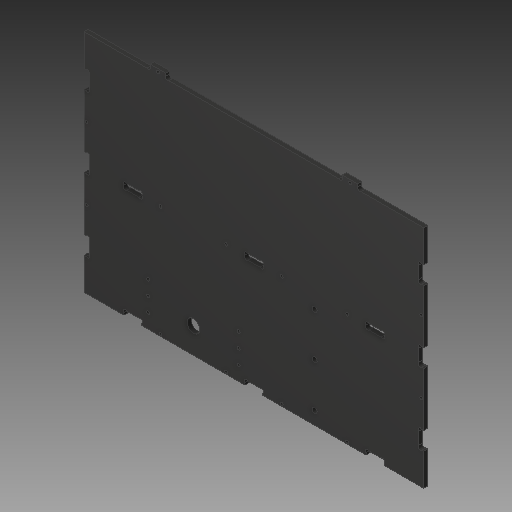
# Autodesk Inventor part: BA02
Saved by Autodesk Inventor 2017 (Build 210142000, 142)
## iProperties
Created: 2019-05-22
Part Number: BA02
Material: Polyethylene, High Density
Document SubType Name: Modeling
Designer: Dell
Density: 0.952 g/cm^3
Appearance: Smooth - Black
Mass: 1090.28 g
Surface Area: 3771.88 cm^2
Volume: 1145.26 cm^3
Author: Dell
Autodesk Inventor part; units mm, degrees
ref_plane "YZ Plane" through (0, 0, 0) normal (1, 0, 0) x (0, 1, 0)
ref_plane "XZ Plane" through (0, 0, 0) normal (0, 1, 0) x (-1, 0, 0)
ref_plane "XY Plane" through (0, 0, 0) normal (0, 0, 1) x (1, 0, 0)
sketch "Sketch1" plane through (0, 0, 0) normal (0, 0, 1) x (1, 0, 0)
  line L0 (0, 0) -> (525.78, 0)
  line L1 (525.78, 0) -> (525.78, 349.25)
  line L2 (525.78, 349.25) -> (0, 349.25)
  line L3 (0, 349.25) -> (0, 0)
  line L4 (239.14, 66.95) -> (239.14, 21.95) construction
  circle A0 centre (239.14, 66.95) radius 2.3813
  circle A1 centre (239.14, 21.95) radius 2.3813
  circle A2 centre (239.14, 44.45) radius 2.3813
  line L5 (179.14, 29.45) -> (179.14, 49.45) construction
  line L6 (169.14, 66.95) -> (169.14, 21.95) construction
  line L7 (179.14, 49.45) -> (159.14, 49.45) construction
  line L8 (159.14, 29.45) -> (179.14, 29.45) construction
  circle A3 centre (169.14, 39.45) radius 10
  line L9 (239.14, 21.95) -> (99.14, 21.95) construction
  line L10 (99.14, 66.95) -> (239.14, 66.95) construction
  line L11 (99.14, 44.45) -> (239.14, 44.45) construction
  line L12 (159.14, 49.45) -> (159.14, 29.45) construction
  line L13 (0, 0) -> (525.78, 0) construction
  line L14 (525.78, 0) -> (525.78, 88.9)
  line L15 (525.78, 88.9) -> (0, 88.9) construction
  line L16 (0, 88.9) -> (0, 0) construction
  line L17 (99.14, 21.95) -> (99.14, 66.95) construction
  circle A4 centre (99.14, 66.95) radius 2.3812
  circle A5 centre (99.14, 21.95) radius 2.3812
  circle A6 centre (99.14, 44.45) radius 2.3812
  point P0 (179.14, 39.45)
  point P1 (159.14, 39.45)
  point P2 (0, 44.45)
  dimension "d0" = 349.25
  dimension "d1" = 525.78
  dimension "d2" = 45
  dimension "d3" = 140
  dimension "d4" = 4.7625
  dimension "d5" = 4.7625
  dimension "d6" = 4.7625
  dimension "d7" = 4.7625
  dimension "d8" = 4.7625
  dimension "d9" = 4.7625
  dimension "d10" = 60
  dimension "d11" = 7.5
  dimension "d12" = 20
  dimension "d13" = 20
  dimension "d15" = 88.9
  dimension "d78" = 169.14
  dimension "d79" = 39.45
  constraints: 36 end point, 8 parallel, 7 midpoint, 6 centre point, 5 coincident, 4 perpendicular, 3 horizontal alignment, 2 horizontal, 2 point on line, 2 other
  measures "d0" distance of L2.end L0.start
  measures "d1" distance of L0.start L0.end
  measures "d2" distance of L4.start L4.end
  measures "d3" distance of L17.end L4.start
  measures "d4" diameter of A4
  measures "d5" diameter of A6
  measures "d6" diameter of A5
  measures "d7" diameter of A1
  measures "d8" diameter of A2
  measures "d9" diameter of A0
  measures "d10" distance from line of L11.end L5
  measures "d11" distance between parallel lines of L9 L8
  measures "d12" distance of L5.end L12.start
  measures "d13" distance of L12.start L8.start
  measures "d15" distance of L15.end L13.start
  measures "d78" distance from line of L3 point (169.14, 39.45)
  measures "d79" distance from line of L0 point (169.14, 39.45)
extrude "Extrusion1" add sketch "Sketch1" along normal blind 6.35
sketch "Sketch2" plane through (0, 0, 6.35) normal (0, 0, 1) x (1, 0, 0)
  line L0 (525.78, 349.25) -> (0, 349.25) projected
  line L1 (101.6, 349.25) -> (127, 349.25)
  line L2 (127, 349.25) -> (127, 355.6)
  line L3 (127, 355.6) -> (101.6, 355.6)
  line L4 (101.6, 355.6) -> (101.6, 349.25)
  line L5 (0, 349.25) -> (0, 0) projected
  line L6 (262.89, 349.25) -> (262.89, 386.8153)
  line L7 (0, 349.25) -> (525.78, 349.25)
  line L8 (424.18, 349.25) -> (398.78, 349.25)
  line L9 (398.78, 349.25) -> (398.78, 355.6)
  line L10 (398.78, 355.6) -> (424.18, 355.6)
  line L11 (424.18, 355.6) -> (424.18, 349.25)
  dimension "d18" = 25.4
  dimension "d19" = 6.35
  dimension "d20" = 101.6
  constraints: 20 end point, 6 symmetric about line, 2 parallel, 2 point on line, 1 horizontal, 1 midpoint, 1 perpendicular, 1 vertical
  measures "d18" distance of L3.end L2.end
  measures "d19" distance of L2.end L1.end
  measures "d20" distance from line of L5 L3.end
extrude "Extrusion2" add sketch "Sketch2" against normal blind 6.35
sketch "Sketch3" plane through (0, 0, 6.35) normal (0, 0, 1) x (1, 0, 0)
  line L0 (101.6, 355.6) -> (101.6, 349.25) projected
  line L1 (127, 355.6) -> (101.6, 355.6) projected
  line L2 (424.18, 355.6) -> (424.18, 349.25) projected
  line L3 (398.78, 355.6) -> (424.18, 355.6) projected
  circle A0 centre (114.3, 352.425) radius 2.25
  circle A1 centre (411.48, 352.425) radius 2.25
  point P0 (0, 0)
  point P1 (114.3, 355.6)
  point P2 (101.6, 352.425)
  point P3 (424.18, 352.425)
  point P4 (411.48, 355.6)
  dimension "d23" = 4.5
  dimension "d24" = 4.5
  constraints: 4 midpoint, 2 centre point, 2 horizontal alignment, 2 vertical alignment
  measures "d23" diameter of A0
  measures "d24" diameter of A1
extrude "Extrusion3" cut sketch "Sketch3" against normal through all
sketch "Sketch4" plane through (0, 0, 6.35) normal (0, 0, 1) x (1, 0, 0)
  line L0 (0, 349.25) -> (0, 0) projected
  line L1 (0, 298.45) -> (6.35, 298.45)
  line L2 (6.35, 298.45) -> (6.35, 273.05)
  line L3 (6.35, 273.05) -> (0, 273.05)
  line L4 (0, 273.05) -> (0, 298.45)
  line L5 (0, 187.325) -> (6.35, 187.325)
  line L6 (6.35, 187.325) -> (6.35, 161.925)
  line L7 (6.35, 161.925) -> (0, 161.925)
  line L8 (0, 161.925) -> (0, 187.325)
  line L9 (0, 50.8) -> (6.35, 50.8)
  line L10 (6.35, 50.8) -> (6.35, 76.2)
  line L11 (6.35, 76.2) -> (0, 76.2)
  line L12 (0, 76.2) -> (0, 50.8)
  line L13 (398.78, 349.25) -> (127, 349.25) projected
  line L14 (262.89, 349.25) -> (262.89, 381.8004)
  line L15 (525.78, 349.25) -> (525.78, 0)
  line L16 (525.78, 298.45) -> (519.43, 298.45)
  line L17 (519.43, 298.45) -> (519.43, 273.05)
  line L18 (519.43, 273.05) -> (525.78, 273.05)
  line L19 (525.78, 273.05) -> (525.78, 298.45)
  line L20 (525.78, 187.325) -> (519.43, 187.325)
  line L21 (519.43, 187.325) -> (519.43, 161.925)
  line L22 (519.43, 161.925) -> (525.78, 161.925)
  line L23 (525.78, 161.925) -> (525.78, 187.325)
  line L24 (525.78, 50.8) -> (519.43, 50.8)
  line L25 (519.43, 50.8) -> (519.43, 76.2)
  line L26 (519.43, 76.2) -> (525.78, 76.2)
  line L27 (525.78, 76.2) -> (525.78, 50.8)
  point P0 (0, 174.625)
  point P1 (525.78, 174.625)
  dimension "d27" = 6.35
  dimension "d28" = 25.4
  dimension "d29" = 6.35
  dimension "d30" = 25.4
  dimension "d31" = 6.35
  dimension "d32" = 25.4
  dimension "d33" = 50.8
  dimension "d34" = 50.8
  constraints: 52 end point, 15 symmetric about line, 6 parallel, 6 point on line, 3 horizontal, 3 midpoint, 3 perpendicular, 1 vertical
  measures "d27" distance of L2.end L3.end
  measures "d28" distance of L1.end L2.end
  measures "d29" distance of L6.end L7.end
  measures "d30" distance of L5.end L6.end
  measures "d31" distance of L11.end L10.end
  measures "d32" distance of L9.end L10.end
  measures "d33" distance from line of L0.start L1
  measures "d34" distance from line of L0.end L9
extrude "Extrusion4" cut sketch "Sketch4" against normal through all
sketch "Sketch5" plane through (0, 0, 0) normal (0, -1, 0) x (1, 0, 0)
  line L0 (62.69, 12.7) -> (88.09, 12.7)
  line L1 (88.09, 12.7) -> (88.09, 0)
  line L2 (88.09, 0) -> (62.69, 0)
  line L3 (62.69, 0) -> (62.69, 12.7)
  line L4 (250.19, 12.7) -> (275.59, 12.7)
  line L5 (275.59, 12.7) -> (275.59, 0)
  line L6 (275.59, 0) -> (250.19, 0)
  line L7 (250.19, 0) -> (250.19, 12.7)
  line L8 (437.69, 12.7) -> (463.09, 12.7)
  line L9 (463.09, 12.7) -> (463.09, 0)
  line L10 (463.09, 0) -> (437.69, 0)
  line L11 (437.69, 0) -> (437.69, 12.7)
  line L12 (75.39, 0) -> (450.39, 0) construction
  line L13 (0, 0) -> (525.78, 0) projected
  point P0 (262.89, 12.7)
  point P1 (262.89, 12.7)
  point P2 (262.89, 0)
  dimension "d37" = 25.4
  dimension "d38" = 12.7
  dimension "d39" = 25.4
  dimension "d40" = 12.7
  dimension "d41" = 25.4
  dimension "d42" = 12.7
  dimension "d43" = 375
  constraints: 26 end point, 6 midpoint, 6 parallel, 3 horizontal, 3 perpendicular, 1 point on line, 1 vertical alignment
  measures "d37" distance of L1.end L2.end
  measures "d38" distance of L1.start L1.end
  measures "d39" distance of L6.start L7.start
  measures "d40" distance of L4.end L6.start
  measures "d41" distance of L9.end L10.end
  measures "d42" distance of L8.end L9.end
  measures "d43" distance of L12.start L12.end
extrude "Extrusion5" cut sketch "Sketch5" against normal blind 6.35
sketch "Sketch6" plane through (0, 0, 6.35) normal (0, 0, 1) x (1, 0, 0)
  line L0 (62.69, 177.325) -> (88.09, 177.325)
  line L1 (88.09, 177.325) -> (88.09, 170.975)
  line L2 (88.09, 170.975) -> (62.69, 170.975)
  line L3 (62.69, 170.975) -> (62.69, 177.325)
  line L4 (250.19, 170.975) -> (275.59, 170.975)
  line L5 (275.59, 170.975) -> (275.59, 177.325)
  line L6 (275.59, 177.325) -> (250.19, 177.325)
  line L7 (250.19, 177.325) -> (250.19, 170.975)
  line L8 (437.69, 170.975) -> (463.09, 170.975)
  line L9 (463.09, 170.975) -> (463.09, 177.325)
  line L10 (463.09, 177.325) -> (437.69, 177.325)
  line L11 (437.69, 177.325) -> (437.69, 170.975)
  line L12 (6.35, 187.325) -> (6.35, 161.925) projected
  line L13 (62.69, 6.35) -> (88.09, 6.35) projected
  line L14 (250.19, 6.35) -> (275.59, 6.35) projected
  line L15 (437.69, 6.35) -> (463.09, 6.35) projected
  point P0 (0, 0)
  dimension "d48" = 6.35
  dimension "d49" = 10
  constraints: 24 end point, 6 parallel, 6 vertical alignment, 3 horizontal, 3 horizontal alignment, 3 perpendicular, 1 point on line
  measures "d48" distance of L0.end L1.end
  measures "d49" distance from line of L12.start L0
extrude "Extrusion6" cut sketch "Sketch6" against normal through all
sketch "Sketch7" plane through (0, 0, 6.35) normal (0, 0, 1) x (1, 0, 0)
  line L0 (275.59, 0) -> (437.69, 0) construction
  line L1 (331.24, 0) -> (382.04, 0) construction
  line L2 (382.04, 0) -> (382.04, 177.325) construction
  line L3 (382.04, 177.325) -> (331.24, 177.325) construction
  line L4 (331.24, 177.325) -> (331.24, 0) construction
  circle A0 centre (356.64, 155.42) radius 4
  circle A1 centre (356.64, 87.71) radius 4
  circle A2 centre (356.64, 20) radius 4
  circle A3 centre (305.84, 174.15) radius 2.25
  circle A4 centre (407.44, 174.15) radius 2.25
  circle A5 centre (305.84, 3.175) radius 2.25
  circle A6 centre (407.44, 3.175) radius 2.25
  line L5 (275.59, 6.35) -> (275.59, 0) projected
  line L6 (437.69, 170.975) -> (437.69, 177.325) projected
  line L7 (262.89, 3.175) -> (305.84, 3.175)
  line L8 (275.59, 0) -> (437.69, 0) projected
  line L9 (250.19, 6.35) -> (275.59, 6.35) projected
  point P0 (0, 0)
  point P1 (275.59, 177.325)
  point P2 (356.64, 0)
  point P3 (356.64, 177.325)
  point P4 (382.04, 88.6625)
  point P5 (275.59, 3.175)
  point P6 (437.69, 174.15)
  point P7 (262.89, 6.35)
  dimension "d50" = 50.8
  dimension "d51" = 8
  dimension "d52" = 8
  dimension "d53" = 8
  dimension "d55" = 20
  dimension "d72" = 4.5
  dimension "d73" = 4.5
  dimension "d74" = 4.5
  dimension "d75" = 4.5
  dimension "d76" = 25.4
  dimension "d77" = 25.4
  dimension "d149" = 67.71
  dimension "d150" = 67.71
  constraints: 10 end point, 7 centre point, 7 midpoint, 6 vertical alignment, 5 horizontal alignment, 3 parallel, 1 horizontal, 1 perpendicular, 1 point on line
  measures "d50" distance of L3.end L2.end
  measures "d51" diameter of A0
  measures "d52" diameter of A1
  measures "d53" diameter of A2
  measures "d55" distance from line of L0 A2.centre
  measures "d72" diameter of A3
  measures "d73" diameter of A4
  measures "d74" diameter of A5
  measures "d75" diameter of A6
  measures "d76" distance from line of A3.centre L4
  measures "d77" distance from line of A4.centre L2
  measures "d149" distance of A0.centre A1.centre
  measures "d150" distance of A2.centre A1.centre
extrude "Extrusion7" cut sketch "Sketch7" against normal through all
sketch "Sketch11" plane through (0, 0, 6.35) normal (0, 0, 1) x (1, 0, 0)
  line L0 (0, 50.8) -> (0, 0) projected
  line L1 (0, 49.53) -> (7.62, 49.53)
  line L2 (7.62, 49.53) -> (7.62, 77.47)
  line L3 (7.62, 77.47) -> (0, 77.47)
  line L4 (0, 77.47) -> (0, 49.53)
  line L5 (0, 161.925) -> (0, 76.2) projected
  line L6 (0, 160.655) -> (7.62, 160.655)
  line L7 (7.62, 160.655) -> (7.62, 188.595)
  line L8 (7.62, 188.595) -> (0, 188.595)
  line L9 (0, 188.595) -> (0, 160.655)
  line L10 (0, 273.05) -> (0, 187.325) projected
  line L11 (0, 271.78) -> (7.62, 271.78)
  line L12 (7.62, 271.78) -> (7.62, 299.72)
  line L13 (7.62, 299.72) -> (0, 299.72)
  line L14 (0, 299.72) -> (0, 271.78)
  line L15 (0, 0) -> (525.78, 0) projected
  line L16 (61.42, 0) -> (89.36, 0)
  line L17 (89.36, 0) -> (89.36, 7.62)
  line L18 (89.36, 7.62) -> (61.42, 7.62)
  line L19 (61.42, 7.62) -> (61.42, 0)
  line L20 (0, 0) -> (525.78, 0) projected
  line L21 (248.92, 0) -> (276.86, 0)
  line L22 (276.86, 0) -> (276.86, 7.62)
  line L23 (276.86, 7.62) -> (248.92, 7.62)
  line L24 (248.92, 7.62) -> (248.92, 0)
  line L25 (275.59, 0) -> (437.69, 0) projected
  line L26 (436.42, 0) -> (464.36, 0)
  line L27 (464.36, 0) -> (464.36, 7.62)
  line L28 (464.36, 7.62) -> (436.42, 7.62)
  line L29 (436.42, 7.62) -> (436.42, 0)
  line L30 (248.92, 169.705) -> (276.86, 169.705)
  line L31 (276.86, 169.705) -> (276.86, 178.595)
  line L32 (276.86, 178.595) -> (248.92, 178.595)
  line L33 (248.92, 178.595) -> (248.92, 169.705)
  line L34 (436.42, 169.705) -> (464.36, 169.705)
  line L35 (464.36, 169.705) -> (464.36, 178.595)
  line L36 (464.36, 178.595) -> (436.42, 178.595)
  line L37 (436.42, 178.595) -> (436.42, 169.705)
  line L38 (525.78, 0) -> (525.78, 50.8) projected
  line L39 (525.78, 49.53) -> (518.16, 49.53)
  line L40 (518.16, 49.53) -> (518.16, 77.47)
  line L41 (518.16, 77.47) -> (525.78, 77.47)
  line L42 (525.78, 77.47) -> (525.78, 49.53)
  line L43 (525.78, 160.655) -> (518.16, 160.655)
  line L44 (518.16, 160.655) -> (518.16, 188.595)
  line L45 (518.16, 188.595) -> (525.78, 188.595)
  line L46 (525.78, 188.595) -> (525.78, 160.655)
  line L47 (525.78, 187.325) -> (525.78, 273.05) projected
  line L48 (525.78, 271.78) -> (518.16, 271.78)
  line L49 (518.16, 271.78) -> (518.16, 299.72)
  line L50 (518.16, 299.72) -> (525.78, 299.72)
  line L51 (525.78, 299.72) -> (525.78, 271.78)
  line L52 (519.43, 50.8) -> (519.43, 76.2) projected
  line L53 (519.43, 161.925) -> (519.43, 187.325) projected
  line L54 (519.43, 273.05) -> (519.43, 298.45) projected
  line L55 (250.19, 170.975) -> (250.19, 177.325) projected
  line L56 (437.69, 170.975) -> (437.69, 177.325) projected
  line L57 (6.35, 187.325) -> (6.35, 161.925) projected
  line L58 (6.35, 76.2) -> (6.35, 50.8) projected
  line L59 (6.35, 298.45) -> (6.35, 273.05) projected
  line L60 (62.69, 6.35) -> (88.09, 6.35) projected
  line L61 (250.19, 6.35) -> (275.59, 6.35) projected
  line L62 (437.69, 6.35) -> (463.09, 6.35) projected
  line L63 (437.69, 177.325) -> (463.09, 177.325) projected
  line L64 (519.43, 187.325) -> (525.78, 187.325) projected
  line L65 (519.43, 76.2) -> (525.78, 76.2) projected
  line L66 (525.78, 273.05) -> (519.43, 273.05) projected
  line L67 (250.19, 0) -> (250.19, 6.35) projected
  line L68 (62.69, 0) -> (62.69, 6.35) projected
  line L69 (275.59, 170.975) -> (250.19, 170.975) projected
  line L70 (61.42, 169.705) -> (89.36, 169.705)
  line L71 (89.36, 169.705) -> (89.36, 178.595)
  line L72 (89.36, 178.595) -> (61.42, 178.595)
  line L73 (61.42, 178.595) -> (61.42, 169.705)
  line L74 (88.09, 170.975) -> (62.69, 170.975) projected
  line L75 (62.69, 170.975) -> (62.69, 177.325) projected
  circle A0 centre (129.2451, 351.4951) radius 3.175
  circle A1 centre (99.3549, 351.4951) radius 3.175
  circle A2 centre (396.5349, 351.4951) radius 3.175
  circle A3 centre (426.4251, 351.4951) radius 3.175
  line L76 (101.6, 349.25) -> (99.3549, 351.4951) construction
  line L77 (101.6, 349.25) -> (101.6, 355.6) projected
  point P0 (88.09, 0)
  point P1 (519.43, 63.5)
  point P2 (518.16, 63.5)
  point P3 (519.43, 174.625)
  point P4 (518.16, 174.625)
  point P5 (519.43, 285.75)
  point P6 (518.16, 285.75)
  point P7 (250.19, 174.15)
  point P8 (248.92, 174.15)
  point P9 (437.69, 174.15)
  point P10 (436.42, 174.15)
  point P11 (6.35, 174.625)
  point P12 (7.62, 174.625)
  point P13 (6.35, 63.5)
  point P14 (7.62, 63.5)
  point P15 (6.35, 285.75)
  point P16 (7.62, 285.75)
  point P17 (75.39, 6.35)
  point P18 (75.39, 7.62)
  point P19 (75.39, 6.35)
  point P20 (262.89, 6.35)
  point P21 (262.89, 7.62)
  point P22 (450.39, 6.35)
  point P23 (450.39, 7.62)
  point P24 (262.89, 170.975)
  point P25 (262.89, 169.705)
  point P26 (75.39, 170.975)
  point P27 (75.39, 169.705)
  point P28 (62.69, 174.15)
  point P29 (61.42, 174.15)
  point P30 (398.78, 349.25)
  point P31 (424.18, 349.25)
  point P32 (127, 349.25)
  dimension "d144" = 6.35
  dimension "d145" = 6.35
  dimension "d146" = 6.35
  dimension "d147" = 6.35
  dimension "d84" = 1.27
  dimension "d85" = 1.27
  dimension "d86" = 1.27
  dimension "d87" = 1.27
  dimension "d88" = 1.27
  dimension "d89" = 1.27
  dimension "d90" = 1.27
  dimension "d91" = 1.27
  dimension "d92" = 1.27
  dimension "d93" = 1.27
  dimension "d94" = 1.27
  dimension "d95" = 1.27
  dimension "d148" = 45
  constraints: 98 end point, 29 midpoint, 24 parallel, 17 point on line, 14 horizontal alignment, 12 horizontal, 12 perpendicular, 9 vertical alignment, 4 coincident, 12 other
  measures "d84" distance between parallel lines of L37 L56
  measures "d85" distance between parallel lines of L36 L63
  measures "d86" distance between parallel lines of L44 L53
  measures "d87" distance between parallel lines of L45 L64
  measures "d88" distance between parallel lines of L41 L65
  measures "d89" distance between parallel lines of L66 L48
  measures "d90" distance between parallel lines of L28 L62
  measures "d91" distance between parallel lines of L24 L67
  measures "d92" distance between parallel lines of L19 L68
  measures "d93" distance between parallel lines of L73 L75
  measures "d94" distance between parallel lines of L70 L74
  measures "d95" distance between parallel lines of L58 L2
  measures "d148" angle of L77 L76
extrude "Extrusion10" cut sketch "Sketch11" against normal through all
sketch "Sketch12" plane through (0, 0, 6.35) normal (0, 0, 1) x (1, 0, 0)
  line L0 (101.6, 355.6) -> (101.6, 349.25) projected
  line L1 (101.6, 355.6) -> (127, 355.6)
  line L2 (127, 355.6) -> (127, 356.87)
  line L3 (127, 356.87) -> (101.6, 356.87)
  line L4 (101.6, 356.87) -> (101.6, 355.6)
  line L5 (398.78, 355.6) -> (424.18, 355.6) projected
  line L6 (398.78, 355.6) -> (424.18, 355.6)
  line L7 (424.18, 355.6) -> (424.18, 356.87)
  line L8 (424.18, 356.87) -> (398.78, 356.87)
  line L9 (398.78, 356.87) -> (398.78, 355.6)
  point P0 (0, 0)
  point P1 (101.6, 347.6625)
  dimension "d132" = 1.27
  constraints: 16 end point, 4 parallel, 2 horizontal, 2 perpendicular, 1 coincident, 1 horizontal alignment
  measures "d132" distance of L3.end L0.start
extrude "Extrusion11" add sketch "Sketch12" against normal up to surface (6.35 mm away) from surface at 0
sketch "Sketch14" plane through (0, 0, 6.35) normal (0, 0, 1) x (1, 0, 0)
  line L0 (101.6, 356.87) -> (127, 356.87) projected
  line L1 (101.6, 356.87) -> (102.235, 356.87)
  line L2 (102.235, 356.87) -> (102.235, 350.1587)
  line L3 (102.235, 350.1587) -> (101.6, 350.1587)
  line L4 (101.6, 350.1587) -> (101.6, 356.87)
  line L5 (127, 356.87) -> (126.365, 356.87)
  line L6 (126.365, 356.87) -> (126.365, 350.1587)
  line L7 (126.365, 350.1587) -> (127, 350.1587)
  line L8 (127, 350.1587) -> (127, 356.87)
  line L9 (398.78, 356.87) -> (424.18, 356.87) projected
  line L10 (398.78, 356.87) -> (399.415, 356.87)
  line L11 (399.415, 356.87) -> (399.415, 350.1587)
  line L12 (399.415, 350.1587) -> (398.78, 350.1587)
  line L13 (398.78, 350.1587) -> (398.78, 356.87)
  line L14 (424.18, 356.87) -> (424.18, 353.7401) projected
  line L15 (424.18, 356.87) -> (423.545, 356.87)
  line L16 (423.545, 356.87) -> (423.545, 350.1587)
  line L17 (423.545, 350.1587) -> (424.18, 350.1587)
  line L18 (424.18, 350.1587) -> (424.18, 356.87)
  arc A0 (97.1099, 349.25) -> (101.6, 353.7401) centre (99.3549, 351.4951) ccw projected
  point P0 (0, 0)
  dimension "d151" = 0.635
  dimension "d152" = 0.635
  dimension "d153" = 0.635
  dimension "d154" = 0.635
  constraints: 32 end point, 8 parallel, 4 horizontal, 4 perpendicular, 3 point on line, 1 point on circle
  measures "d151" distance between parallel lines of L13 L11
  measures "d152" distance between parallel lines of L14 L16
  measures "d153" distance between parallel lines of L8 L6
  measures "d154" distance between parallel lines of L4 L2
extrude "Extrusion12" cut sketch "Sketch14" against normal through all contours L0 L2 A0 L4 | A0 L2 L3 L4 | L0 L8 L7 L6 | L9 L11 L12 L13 | L9 L14 L18 L17 L16
sketch "Sketch15" plane through (0, 0, 6.35) normal (0, 0, 1) x (1, 0, 0)
  circle A0 centre (239.14, 66.95) radius 2.3813 construction
  circle A1 centre (239.14, 44.45) radius 2.3813 construction
  circle A2 centre (239.14, 21.95) radius 2.3813 construction
  circle A3 centre (99.14, 21.95) radius 2.3812 construction
  circle A4 centre (99.14, 44.45) radius 2.3812 construction
  circle A5 centre (99.14, 66.95) radius 2.3812 construction
  circle A6 centre (169.14, 39.45) radius 10 construction
  circle A7 centre (411.48, 352.425) radius 2.25 construction
  circle A8 centre (114.3, 352.425) radius 2.25 construction
  circle A9 centre (356.64, 20) radius 4 construction
  circle A10 centre (356.64, 155.42) radius 4 construction
  circle A11 centre (305.84, 3.175) radius 2.25 construction
  circle A12 centre (305.84, 174.15) radius 2.25 construction
  circle A13 centre (407.44, 174.15) radius 2.25 construction
  circle A14 centre (407.44, 3.175) radius 2.25 construction
  circle A15 centre (356.64, 87.71) radius 4 construction
  line L0 (89.36, 178.595) -> (89.36, 169.705) construction
  line L1 (89.36, 169.705) -> (61.42, 169.705) construction
  line L2 (61.42, 169.705) -> (61.42, 178.595) construction
  line L3 (61.42, 178.595) -> (89.36, 178.595) construction
  line L4 (464.36, 178.595) -> (464.36, 169.705) construction
  line L5 (464.36, 169.705) -> (436.42, 169.705) construction
  line L6 (436.42, 169.705) -> (436.42, 178.595) construction
  line L7 (436.42, 178.595) -> (464.36, 178.595) construction
  line L8 (276.86, 178.595) -> (276.86, 169.705) construction
  line L9 (276.86, 169.705) -> (248.92, 169.705) construction
  line L10 (248.92, 169.705) -> (248.92, 178.595) construction
  line L11 (248.92, 178.595) -> (276.86, 178.595) construction
  line L12 (399.415, 356.87) -> (399.415, 352.8314) construction
  arc A16 (394.2899, 349.25) -> (399.415, 352.8314) centre (396.5349, 351.4951) ccw construction
  line L13 (394.2899, 349.25) -> (131.4901, 349.25) construction
  arc A17 (126.365, 352.8314) -> (131.4901, 349.25) centre (129.2451, 351.4951) ccw construction
  line L14 (126.365, 352.8314) -> (126.365, 356.87) construction
  line L15 (102.235, 356.87) -> (126.365, 356.87) construction
  line L16 (102.235, 356.87) -> (102.235, 352.8314) construction
  arc A18 (97.1099, 349.25) -> (102.235, 352.8314) centre (99.3549, 351.4951) ccw construction
  line L17 (97.1099, 349.25) -> (0, 349.25) construction
  line L18 (0, 349.25) -> (0, 299.72) construction
  line L19 (0, 299.72) -> (7.62, 299.72) construction
  line L20 (7.62, 299.72) -> (7.62, 271.78) construction
  line L21 (7.62, 271.78) -> (0, 271.78) construction
  line L22 (0, 271.78) -> (0, 188.595) construction
  line L23 (0, 188.595) -> (7.62, 188.595) construction
  line L24 (7.62, 188.595) -> (7.62, 160.655) construction
  line L25 (7.62, 160.655) -> (0, 160.655) construction
  line L26 (0, 160.655) -> (0, 77.47) construction
  line L27 (0, 77.47) -> (7.62, 77.47) construction
  line L28 (7.62, 77.47) -> (7.62, 49.53) construction
  line L29 (7.62, 49.53) -> (0, 49.53) construction
  line L30 (0, 49.53) -> (0, 0) construction
  line L31 (0, 0) -> (61.42, 0) construction
  line L32 (61.42, 0) -> (61.42, 7.62) construction
  line L33 (61.42, 7.62) -> (89.36, 7.62) construction
  line L34 (89.36, 7.62) -> (89.36, 0) construction
  line L35 (89.36, 0) -> (248.92, 0) construction
  line L36 (248.92, 0) -> (248.92, 7.62) construction
  line L37 (248.92, 7.62) -> (276.86, 7.62) construction
  line L38 (276.86, 7.62) -> (276.86, 0) construction
  line L39 (276.86, 0) -> (436.42, 0) construction
  line L40 (436.42, 0) -> (436.42, 7.62) construction
  line L41 (436.42, 7.62) -> (464.36, 7.62) construction
  line L42 (464.36, 7.62) -> (464.36, 0) construction
  line L43 (464.36, 0) -> (525.78, 0) construction
  line L44 (525.78, 0) -> (525.78, 49.53) construction
  line L45 (525.78, 49.53) -> (518.16, 49.53) construction
  line L46 (518.16, 49.53) -> (518.16, 77.47) construction
  line L47 (518.16, 77.47) -> (525.78, 77.47) construction
  line L48 (525.78, 77.47) -> (525.78, 160.655) construction
  line L49 (525.78, 160.655) -> (518.16, 160.655) construction
  line L50 (518.16, 160.655) -> (518.16, 188.595) construction
  line L51 (518.16, 188.595) -> (525.78, 188.595) construction
  line L52 (525.78, 188.595) -> (525.78, 271.78) construction
  line L53 (525.78, 271.78) -> (518.16, 271.78) construction
  line L54 (518.16, 271.78) -> (518.16, 299.72) construction
  line L55 (518.16, 299.72) -> (525.78, 299.72) construction
  line L56 (525.78, 299.72) -> (525.78, 349.25) construction
  line L57 (525.78, 349.25) -> (428.6701, 349.25) construction
  arc A19 (423.545, 352.8314) -> (428.6701, 349.25) centre (426.4251, 351.4951) ccw construction
  line L58 (423.545, 352.8314) -> (423.545, 356.87) construction
  line L59 (399.415, 356.87) -> (423.545, 356.87) construction
  line L60 (87.1149, 5.3749) -> (63.6651, 5.3749) construction
  line L61 (63.6651, 5.3749) -> (63.6651, -2.2451) construction
  line L62 (63.6651, -2.2451) -> (-2.2451, -2.2451) construction
  line L63 (-2.2451, -2.2451) -> (-2.2451, 51.7751) construction
  line L64 (-2.2451, 51.7751) -> (5.3749, 51.7751) construction
  line L65 (5.3749, 51.7751) -> (5.3749, 75.2249) construction
  line L66 (5.3749, 75.2249) -> (-2.2451, 75.2249) construction
  line L67 (-2.2451, 75.2249) -> (-2.2451, 162.9001) construction
  line L68 (-2.2451, 162.9001) -> (5.3749, 162.9001) construction
  line L69 (5.3749, 162.9001) -> (5.3749, 186.3499) construction
  line L70 (5.3749, 186.3499) -> (-2.2451, 186.3499) construction
  line L71 (-2.2451, 186.3499) -> (-2.2451, 274.0251) construction
  line L72 (-2.2451, 274.0251) -> (5.3749, 274.0251) construction
  line L73 (5.3749, 274.0251) -> (5.3749, 297.4749) construction
  line L74 (5.3749, 297.4749) -> (-2.2451, 297.4749) construction
  line L75 (-2.2451, 297.4749) -> (-2.2451, 351.4951) construction
  line L76 (-2.2451, 351.4951) -> (99.9899, 351.4951) construction
  line L77 (99.9899, 351.4951) -> (99.9899, 359.1151) construction
  line L78 (99.9899, 359.1151) -> (128.6101, 359.1151) construction
  line L79 (128.6101, 359.1151) -> (128.6101, 351.4951) construction
  line L80 (128.6101, 351.4951) -> (397.1699, 351.4951) construction
  line L81 (397.1699, 351.4951) -> (397.1699, 359.1151) construction
  line L82 (397.1699, 359.1151) -> (425.7901, 359.1151) construction
  line L83 (425.7901, 359.1151) -> (425.7901, 351.4951) construction
  line L84 (425.7901, 351.4951) -> (528.0251, 351.4951) construction
  line L85 (528.0251, 351.4951) -> (528.0251, 297.4749) construction
  line L86 (528.0251, 297.4749) -> (520.4051, 297.4749) construction
  line L87 (520.4051, 297.4749) -> (520.4051, 274.0251) construction
  line L88 (520.4051, 274.0251) -> (528.0251, 274.0251) construction
  line L89 (528.0251, 274.0251) -> (528.0251, 186.3499) construction
  line L90 (528.0251, 186.3499) -> (520.4051, 186.3499) construction
  line L91 (520.4051, 186.3499) -> (520.4051, 162.9001) construction
  line L92 (520.4051, 162.9001) -> (528.0251, 162.9001) construction
  line L93 (528.0251, 162.9001) -> (528.0251, 75.2249) construction
  line L94 (528.0251, 75.2249) -> (520.4051, 75.2249) construction
  line L95 (520.4051, 75.2249) -> (520.4051, 51.7751) construction
  line L96 (520.4051, 51.7751) -> (528.0251, 51.7751) construction
  line L97 (528.0251, 51.7751) -> (528.0251, -2.2451) construction
  line L98 (528.0251, -2.2451) -> (462.1149, -2.2451) construction
  line L99 (462.1149, -2.2451) -> (462.1149, 5.3749) construction
  line L100 (462.1149, 5.3749) -> (438.6651, 5.3749) construction
  line L101 (438.6651, 5.3749) -> (438.6651, -2.2451) construction
  line L102 (438.6651, -2.2451) -> (274.6149, -2.2451) construction
  line L103 (274.6149, -2.2451) -> (274.6149, 5.3749) construction
  line L104 (274.6149, 5.3749) -> (251.1651, 5.3749) construction
  line L105 (251.1651, 5.3749) -> (251.1651, -2.2451) construction
  line L106 (251.1651, -2.2451) -> (87.1149, -2.2451) construction
  line L107 (87.1149, -2.2451) -> (87.1149, 5.3749) construction
  line L108 (87.1149, 176.3499) -> (87.1149, 171.9501) construction
  line L109 (87.1149, 171.9501) -> (63.6651, 171.9501) construction
  line L110 (63.6651, 171.9501) -> (63.6651, 176.3499) construction
  line L111 (63.6651, 176.3499) -> (87.1149, 176.3499) construction
  line L112 (274.6149, 176.3499) -> (274.6149, 171.9501) construction
  line L113 (274.6149, 171.9501) -> (251.1651, 171.9501) construction
  line L114 (251.1651, 171.9501) -> (251.1651, 176.3499) construction
  line L115 (251.1651, 176.3499) -> (274.6149, 176.3499) construction
  line L116 (462.1149, 176.3499) -> (462.1149, 171.9501) construction
  line L117 (462.1149, 171.9501) -> (438.6651, 171.9501) construction
  line L118 (438.6651, 171.9501) -> (438.6651, 176.3499) construction
  line L119 (438.6651, 176.3499) -> (462.1149, 176.3499) construction
  circle A20 centre (63.6651, 5.3749) radius 3.175
  circle A21 centre (87.1149, 5.3749) radius 3.175
  line L120 (7.62, 77.47) -> (0, 77.47) projected
  circle A22 centre (5.3749, 75.2249) radius 3.175
  circle A23 centre (5.3749, 51.7751) radius 3.175
  circle A24 centre (5.3749, 162.9001) radius 3.175
  line L121 (7.62, 188.595) -> (0, 188.595) projected
  circle A25 centre (5.3749, 186.3499) radius 3.175
  circle A26 centre (5.3749, 297.4749) radius 3.175
  circle A27 centre (5.3749, 274.0251) radius 3.175
  circle A28 centre (520.4051, 297.4749) radius 3.175
  circle A29 centre (520.4051, 274.0251) radius 3.175
  circle A30 centre (520.4051, 186.3499) radius 3.175
  circle A31 centre (520.4051, 162.9001) radius 3.175
  circle A32 centre (520.4051, 75.2249) radius 3.175
  circle A33 centre (520.4051, 51.7751) radius 3.175
  circle A34 centre (462.1149, 5.3749) radius 3.175
  circle A35 centre (438.6651, 5.3749) radius 3.175
  line L122 (276.86, 7.62) -> (248.92, 7.62) projected
  circle A36 centre (251.1651, 5.3749) radius 3.175
  circle A37 centre (274.6149, 5.3749) radius 3.175
  circle A38 centre (462.1149, 176.3499) radius 3.175
  circle A39 centre (462.1149, 171.9501) radius 3.175
  circle A40 centre (438.6651, 171.9501) radius 3.175
  circle A41 centre (438.6651, 176.3499) radius 3.175
  line L123 (276.86, 178.595) -> (276.86, 169.705) projected
  circle A42 centre (274.6149, 176.3499) radius 3.175
  circle A43 centre (274.6149, 171.9501) radius 3.175
  circle A44 centre (251.1651, 171.9501) radius 3.175
  circle A45 centre (251.1651, 176.3499) radius 3.175
  circle A46 centre (87.1149, 176.3499) radius 3.175
  circle A47 centre (87.1149, 171.9501) radius 3.175
  circle A48 centre (63.6651, 176.3499) radius 3.175
  circle A49 centre (63.6651, 171.9501) radius 3.175
  dimension "d157" = 6.35
  dimension "d158" = 6.35
  dimension "d159" = 6.35
  dimension "d160" = 6.35
  constraints: 120 end point, 30 coincident, 146 other
extrude "Extrusion13" cut sketch "Sketch15" against normal through all
sketch "Sketch16" plane through (0, 0, 6.35) normal (0, 0, 1) x (1, 0, 0)
  circle A0 centre (521.97, 230.1875) radius 2.25
  circle A1 centre (521.97, 119.0625) radius 2.25
  line L0 (525.78, 188.595) -> (525.78, 271.78) projected
  line L1 (525.78, 77.47) -> (525.78, 160.655) projected
  circle A2 centre (305.84, 174.15) radius 2.25 projected
  circle A3 centre (407.44, 174.15) radius 2.25 projected
  circle A4 centre (407.44, 3.175) radius 2.25 projected
  circle A5 centre (305.84, 3.175) radius 2.25 projected
  line L2 (272.3699, 7.62) -> (253.4101, 7.62) projected
  line L3 (262.89, 7.62) -> (262.89, -57.6446)
  circle A6 centre (3.81, 230.1875) radius 2.25
  circle A7 centre (3.81, 119.0625) radius 2.25
  line L4 (0, 188.595) -> (0, 271.78)
  line L5 (0, 77.47) -> (0, 160.655)
  circle A8 centre (219.94, 174.15) radius 2.25
  circle A9 centre (118.34, 174.15) radius 2.25
  circle A10 centre (118.34, 3.175) radius 2.25
  circle A11 centre (219.94, 3.175) radius 2.25
  point P0 (0, 0)
  point P1 (525.78, 230.1875)
  point P2 (525.78, 119.0625)
  point P3 (0, 230.1875)
  point P4 (0, 119.0625)
  dimension "d163" = 4.5
  dimension "d164" = 4.5
  dimension "d165" = 3.81
  dimension "d166" = 3.81
  constraints: 12 symmetric about line, 8 centre point, 6 end point, 3 midpoint, 2 horizontal alignment, 1 vertical, 6 other
  measures "d163" diameter of A0
  measures "d164" diameter of A1
  measures "d165" distance from line of L0 A0.centre
  measures "d166" distance from line of L1 A1.centre
extrude "Extrusion14" cut sketch "Sketch16" against normal through all
equation "\"d16\" = Panel_Thickness"
equation "\"d19\" = Panel_Thickness"
equation "\"d21\" = Panel_Thickness"
equation "\"d27\" = Panel_Thickness"
equation "\"d29\" = Panel_Thickness"
equation "\"d31\" = Panel_Thickness"
equation "\"d40\" = d38"
equation "\"d42\" = d40"
equation "\"d44\" = Panel_Thickness"
equation "\"d48\" = Panel_Thickness"
equation "\"d144\" = Tool_Dia"
equation "\"d145\" = Tool_Dia"
equation "\"d146\" = Tool_Dia"
equation "\"d147\" = Tool_Dia"
equation "\"d84\" = Fit_Tolerance"
equation "\"d85\" = Fit_Tolerance"
equation "\"d86\" = Fit_Tolerance"
equation "\"d87\" = Fit_Tolerance"
equation "\"d88\" = Fit_Tolerance"
equation "\"d89\" = Fit_Tolerance"
equation "\"d90\" = Fit_Tolerance"
equation "\"d91\" = Fit_Tolerance"
equation "\"d92\" = Fit_Tolerance"
equation "\"d93\" = Fit_Tolerance"
equation "\"d94\" = Fit_Tolerance"
equation "\"d95\" = Fit_Tolerance"
equation "\"d132\" = Fit_Tolerance"
equation "\"d151\" = 0.5 * Fit_Tolerance"
equation "\"d152\" = 0.5 * Fit_Tolerance"
equation "\"d153\" = 0.5 * Fit_Tolerance"
equation "\"d154\" = 0.5 * Fit_Tolerance"
equation "\"d157\" = Tool_Dia"
equation "\"d158\" = Tool_Dia"
equation "\"d159\" = Tool_Dia"
equation "\"d160\" = Tool_Dia"
equation "\"Fit_Tolerance\" = 1.27"
equation "\"Panel_Thickness\" = 6.35"
equation "\"Tool_Dia\" = 6.35"
body "Solid1"
